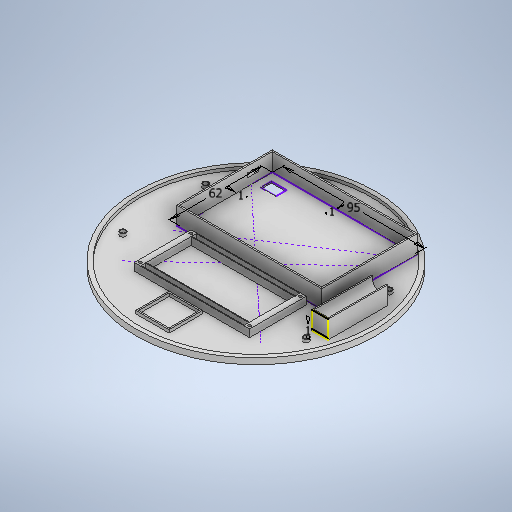
# Autodesk Inventor part: base
Saved by Autodesk Inventor 2025.2 (Build 292293000, 293)
## iProperties
Created: 2026-03-17
Part Number: base
Material: Genérico
Document SubType Name: Modeling
Designer: Periscopio
Density: 1 g/cm^3
Appearance: Valor por defecto
Author: Periscopio
Autodesk Inventor part; units mm, degrees
ref_plane "YZ Plane" through (0, 0, 0) normal (1, 0, 0) x (0, 1, 0)
ref_plane "XZ Plane" through (0, 0, 0) normal (0, 1, 0) x (-1, 0, 0)
ref_plane "XY Plane" through (0, 0, 0) normal (0, 0, 1) x (1, 0, 0)
sketch "Boceto1" plane through (0, 0, 0) normal (0, 1, 0) x (-1, 0, 0)
  circle A0 centre (0, 0) radius 80
  circle A1 centre (0, 0) radius 77.161
  dimension "d0" = 160
  dimension "d6" = 2.839
  constraints: 2 centre point, 2 coincident
  measures "d0" diameter of A0
  measures "d6" radial gap between concentric circles of A0 A1
extrude "Extrusión3" add sketch "Boceto1" along normal blind 4
extrude "Extrusión4" add sketch "Boceto1" along normal blind 2 contours A1
sketch "Boceto2" plane through (0, 2, 0) normal (0, 1, 0) x (1, 0, 0)
  line L0 (47.5, -3.5651) -> (-47.5, -3.5651)
  line L1 (-47.5, -3.5651) -> (-47.5, 58.4349)
  line L2 (-47.5, 58.4349) -> (47.5, 58.4349)
  line L3 (47.5, 58.4349) -> (47.5, -3.5651)
  line L4 (47.5, -44.1835) -> (-47.5, 44.1835) construction
  line L5 (-47.5, -44.1835) -> (47.5, 44.1835) construction
  line L6 (-48.5, -4.5651) -> (48.5, -4.5651)
  line L7 (48.5, -4.5651) -> (48.5, 59.4349)
  line L8 (48.5, 59.4349) -> (-48.5, 59.4349)
  line L9 (-48.5, 59.4349) -> (-48.5, -4.5651)
  line L10 (-48.5, -9.337) -> (48.5, 54.663) construction
  line L11 (48.5, -45.1835) -> (-48.5, 45.1835) construction
  line L12 (-32.3907, 52.8953) -> (-42.5753, 52.8953)
  line L13 (-42.5753, 52.8953) -> (-42.5753, 45.7711)
  line L14 (-42.5753, 45.7711) -> (-32.3907, 45.7711)
  line L15 (-32.3907, 45.7711) -> (-32.3907, 52.8953)
  point P0 (0, 0)
  dimension "d11" = 95
  dimension "d12" = 62
  dimension "d16" = 1
  dimension "d17" = 1
  constraints: 32 end point, 6 parallel, 3 horizontal, 3 midpoint, 3 perpendicular
  measures "d11" distance of L1.end L2.end
  measures "d12" distance of L0.end L1.end
  measures "d16" distance between parallel lines of L2 L8
  measures "d17" distance between parallel lines of L1 L9
extrude "Extrusión5" add sketch "Boceto2" along normal blind 12 contours L9 L8 L7 L6
sketch "Boceto4" plane through (-48.5, 2, -59.4349) normal (-1, 0, 0) x (0, 0, 1)
  line L0 (0, 0) -> (0, 12) projected
  line L1 (0, 12) -> (0, 1.9732)
  line L2 (10, 5.0938) -> (17.4, 5.0938)
  line L3 (17.4, 5.0938) -> (17.4, 7.7938)
  line L4 (17.4, 7.7938) -> (10, 7.7938)
  line L5 (10, 7.7938) -> (10, 5.0938)
  line L6 (10, 5.0938) -> (17.4, 7.7938) construction
  line L7 (17.4, 5.0938) -> (10, 7.7938) construction
  line L8 (9, 4.0938) -> (18.4, 4.0938)
  line L9 (18.4, 4.0938) -> (18.4, 8.7938)
  line L10 (18.4, 8.7938) -> (9, 8.7938)
  line L11 (9, 8.7938) -> (9, 4.0938)
  line L12 (9, 4.0938) -> (18.4, 8.7938) construction
  line L13 (18.4, 4.0938) -> (9, 8.7938) construction
  point P0 (59.4349, -2)
  point P1 (13.7, 6.4438)
  dimension "d22" = 7.4
  dimension "d23" = 2.7
  dimension "d24" = 1
  dimension "d25" = 1
  constraints: 26 end point, 4 parallel, 3 midpoint, 2 horizontal, 2 perpendicular, 1 point on line
  measures "d22" distance of L4.end L3.end
  measures "d23" distance of L3.end L2.end
  measures "d24" distance between parallel lines of L4 L10
  measures "d25" distance between parallel lines of L5 L11
extrude "Extrusión6" cut sketch "Boceto4" against normal blind 14 contours L5 L4 L3 L2
extrude "Extrusión7" add sketch "Boceto4" along normal blind 1
sketch "Boceto6" plane through (0, 2, 0) normal (0, 1, 0) x (1, 0, 0)
  line L0 (-32.4424, -11.0569) -> (36.7172, -11.0569)
  line L1 (36.7172, -11.0569) -> (36.7172, -41.0069)
  line L2 (36.7172, -41.0069) -> (-32.4424, -41.0069)
  line L3 (-32.4424, -41.0069) -> (-32.4424, -11.0569)
  line L4 (-36.4424, -7.0569) -> (40.7172, -7.0569)
  line L5 (40.7172, -7.0569) -> (40.7172, -45.0069)
  line L6 (40.7172, -45.0069) -> (-36.4424, -45.0069)
  line L7 (-36.4424, -45.0069) -> (-36.4424, -7.0569)
  line L8 (36.7172, -7.5569) -> (-32.4424, -7.5569)
  line L9 (-32.4424, -7.5569) -> (-32.4424, -10.5569)
  line L10 (-32.4424, -10.5569) -> (36.7172, -10.5569)
  line L11 (36.7172, -10.5569) -> (36.7172, -7.5569)
  line L12 (36.7172, -44.5069) -> (-32.4424, -44.5069)
  line L13 (-32.4424, -44.5069) -> (-32.4424, -41.5069)
  line L14 (-32.4424, -41.5069) -> (36.7172, -41.5069)
  line L15 (36.7172, -41.5069) -> (36.7172, -44.5069)
  circle A0 centre (38.7172, -9.0569) radius 1
  circle A1 centre (38.7172, -43.0069) radius 1
  circle A2 centre (-34.4424, -9.0569) radius 1
  circle A3 centre (-34.4424, -43.0069) radius 1
  point P0 (0, 0)
  dimension "d32" = 4
  dimension "d41" = 3
  dimension "d42" = 0.5
  dimension "d43" = 2
  constraints: 32 end point, 6 parallel, 4 centre point, 3 horizontal, 3 perpendicular
  measures "d32" distance between parallel lines of L5 L1
  measures "d41" distance between parallel lines of L10 L8
  measures "d42" distance between parallel lines of L0 L10
  measures "d43" diameter of A0
sketch "Boceto7" plane through (0, 2, 0) normal (0, 1, 0) x (1, 0, 0)
  line L0 (-10.16, -47.9931) -> (10.16, -47.9931)
  line L1 (10.16, -47.9931) -> (10.16, -68.3131)
  line L2 (10.16, -68.3131) -> (-10.16, -68.3131)
  line L3 (-10.16, -68.3131) -> (-10.16, -47.9931)
  line L4 (-10.16, -47.9931) -> (10.16, -68.3131) construction
  line L5 (10.16, -47.9931) -> (-10.16, -68.3131) construction
  line L6 (-11.16, -46.9931) -> (11.16, -46.9931)
  line L7 (11.16, -46.9931) -> (11.16, -69.3131)
  line L8 (11.16, -69.3131) -> (-11.16, -69.3131)
  line L9 (-11.16, -69.3131) -> (-11.16, -46.9931)
  line L10 (-11.16, -46.9931) -> (11.16, -69.3131) construction
  line L11 (11.16, -46.9931) -> (-11.16, -69.3131) construction
  point P0 (0, 0)
  point P1 (0, -58.1531)
  dimension "d34" = 20.32
  dimension "d35" = 20.32
  dimension "d36" = 22.32
  dimension "d37" = 22.32
  constraints: 24 end point, 4 midpoint, 4 parallel, 2 horizontal, 2 perpendicular
  measures "d34" distance of L1.end L2.end
  measures "d35" distance of L0.end L1.end
  measures "d36" distance of L7.end L8.end
  measures "d37" distance of L6.end L7.end
extrude "Extrusión8" add sketch "Boceto7" along normal blind 2
extrude "Extrusión9" add sketch "Boceto6" along normal blind 5
thread "Rosca1" size "M2x0.4" class "6H" standard "ANSI Metric M Profile" full length
thread "Rosca2" size "M2x0.4" class "6H" standard "ANSI Metric M Profile" full length
thread "Rosca3" size "M2x0.4" class "6H" standard "ANSI Metric M Profile" full length
thread "Rosca4" size "M2x0.4" class "6H" standard "ANSI Metric M Profile" full length
extrude "Extrusión10" cut sketch "Boceto2" against normal through all contours L15 L14 L13 L12
sketch "Boceto8" plane through (0, 0, 0) normal (0, -1, 0) x (1, 0, 0)
  line L0 (-42.5753, -52.8953) -> (-32.3907, -52.8953) projected
  line L1 (-32.3907, -52.8953) -> (-32.3907, -45.7711) projected
  line L2 (-31.3907, -53.8953) -> (-43.5753, -53.8953)
  line L3 (-43.5753, -53.8953) -> (-43.5753, -44.7711)
  line L4 (-43.5753, -44.7711) -> (-31.3907, -44.7711)
  line L5 (-31.3907, -44.7711) -> (-31.3907, -53.8953)
  line L6 (-31.3907, -53.8953) -> (-43.5753, -44.7711) construction
  line L7 (-43.5753, -53.8953) -> (-31.3907, -44.7711) construction
  line L8 (-42.5753, -52.8953) -> (-42.5753, -45.7711) projected
  line L9 (-42.5753, -52.8953) -> (-32.3907, -52.8953)
  line L10 (-32.3907, -52.8953) -> (-32.3907, -45.7711)
  line L11 (-32.3907, -45.7711) -> (-42.5753, -45.7711)
  line L12 (-42.5753, -45.7711) -> (-42.5753, -52.8953)
  point P0 (0, 0)
  point P1 (-37.483, -49.3332)
  point P2 (-37.483, -52.8953)
  dimension "d56" = 1
  dimension "d57" = 1
  constraints: 20 end point, 4 parallel, 3 midpoint, 2 horizontal, 2 perpendicular
  measures "d56" distance between parallel lines of L8 L3
  measures "d57" distance from line of point (-37.483, -52.895) L2
extrude "Extrusión11" cut sketch "Boceto8" against normal blind 1
sketch "Boceto9" plane through (0, 2, 0) normal (0, 1, 0) x (1, 0, 0)
  circle A0 centre (0, 0) radius 77.161 projected
  line L0 (77.161, 0) -> (48.5, 0)
  line L1 (48.5, 59.4349) -> (48.5, -4.5651) projected
  line L2 (57.3305, 20) -> (68.3305, 20)
  line L3 (68.3305, 20) -> (68.3305, -20)
  line L4 (68.3305, -20) -> (57.3305, -20)
  line L5 (57.3305, -20) -> (57.3305, 20)
  line L6 (57.3305, 20) -> (68.3305, -20) construction
  line L7 (68.3305, 20) -> (57.3305, -20) construction
  point P0 (62.8305, 0)
  dimension "d60" = 11
  dimension "d61" = 40
  constraints: 14 end point, 3 midpoint, 2 horizontal, 2 parallel, 1 horizontal alignment, 1 perpendicular, 1 point on line, 1 other
  measures "d60" distance of L3.end L4.end
  measures "d61" distance of L2.end L3.end
extrude "Extrusión12" add sketch "Boceto9" along normal blind 12 contours L3 L4 L5 L0 | L0 L5 L2 L3
sketch "Boceto11" plane through (57.3305, 2, 20) normal (0, 0, 1) x (1, 0, 0)
  line L0 (11, 0) -> (0, 0) projected
  line L1 (0, 0) -> (0, 1)
  line L2 (0, 0) -> (0, 12) projected
  line L3 (0, 1) -> (11, 1)
  line L4 (11, 0) -> (11, 12) projected
  line L5 (0, 12) -> (11, 12) projected
  line L6 (0, 12) -> (0.5, 12)
  line L7 (11, 12) -> (10.5, 12)
  line L8 (10.167, 12) -> (0.833, 12)
  line L9 (0, 0) -> (11, 0) projected
  line L10 (0, 0) -> (0, 12) projected
  line L11 (11, 12) -> (0, 12) projected
  line L12 (11, 0) -> (11, 12) projected
  point P0 (-57.3305, -2)
  dimension "d64" = 1
  constraints: 10 end point, 6 point on line, 1 collinear, 1 perpendicular
  measures "d64" distance of L0.end L1.end
sketch "Boceto12" plane through (68.3305, 2, -20) normal (0, 0, -1) x (-1, 0, 0)
  arc A0 (0.833, 12) -> (10.167, 12) centre (5.5, 10.2059) ccw projected
  arc A1 (0.5311, 10.7631) -> (10.167, 12) centre (5.4899, 10.2844) ccw
  line L0 (0.833, 12) -> (10.167, 12)
  line L1 (11, 0) -> (11, 12) projected
  point P0 (68.3305, -2)
  constraints: 4 point on circle, 2 end point, 1 centre point, 1 perpendicular
extrude "Extrusión14" cut sketch "Boceto12" against normal blind 39 contours L0 A1 A0
sketch "Boceto13" plane through (0, 2, 0) normal (0, 1, 0) x (1, 0, 0)
  circle A0 centre (-61.3337, 27.7224) radius 1.5
  circle A1 centre (0, 0) radius 77.161 projected
  circle A2 centre (-61.3337, 27.7224) radius 2
  circle A3 centre (-61.3337, -27.7224) radius 1.5
  circle A4 centre (-61.3337, -27.7224) radius 2
  circle A5 centre (61.3337, 27.7224) radius 1.5
  circle A6 centre (61.3337, 27.7224) radius 2
  circle A7 centre (61.3337, -27.7224) radius 2
  circle A8 centre (61.3337, -27.7224) radius 1.5
  line L0 (-61.3337, -27.7224) -> (0, -27.7224)
  line L1 (0, -27.7224) -> (0, 0)
  dimension "d72" = 3
  dimension "d73" = 4
  dimension "d78" = 27.7224
  dimension "d79" = 61.3337
  constraints: 8 centre point, 4 coincident, 4 end point, 1 horizontal, 1 perpendicular
  measures "d72" diameter of A0
  measures "d73" diameter of A2
  measures "d78" distance of L0.end L1.end
  measures "d79" distance of L0.start L0.end
extrude "Extrusión15" add sketch "Boceto13" along normal blind 2 contours A2 | A4 | A6 | A7
extrude "Extrusión16" cut sketch "Boceto13" against normal blind 2 contours A0 | A3 | A5 | A8
